Autodesk Inventor part; units mm, degrees
(part 3 of 18)
  ellipse E264 centre (-10091.4826, -10019.097) end of major axis (-10091.4826, -10024.058) minor radius 0.4679 (-10091.8131, -10015.5852) -> (-10091.9034, -10016.9265) ccw
  ellipse E265 centre (-10091.4826, -10019.097) end of major axis (-10091.4826, -10024.058) minor radius 0.4679 (-10091.9034, -10021.2675) -> (-10091.8131, -10022.6088) ccw
  spline S10 degree 3 poles (-10091.8131, -10022.6088) (-10091.7949, -10022.6489) (-10091.7591, -10022.7279) (-10091.7082, -10022.8453) (-10091.6607, -10022.9592) (-10091.617, -10023.0692) (-10091.5772, -10023.1748) (-10091.5414, -10023.2762) (-10091.5097, -10023.3737) (-10091.4825, -10023.4669) (-10091.4604, -10023.5539) (-10091.4445, -10023.6326) (-10091.435, -10023.7014) (-10091.4315, -10023.7595) (-10091.4337, -10023.8077) (-10091.4421, -10023.8464) (-10091.4557, -10023.8779) (-10091.4713, -10023.8914) (-10091.4786, -10023.8977) knots 0 0 0 0 0.096483 0.190064 0.280343 0.366935 0.449463 0.527566 0.602572 0.674179 0.740358 0.79923 0.84998 0.89243 0.926709 0.955226 0.979191 1 1 1 1
  spline S11 degree 3 poles (-10091.4786, -10014.2963) (-10091.4715, -10014.3024) (-10091.4562, -10014.3157) (-10091.4427, -10014.3469) (-10091.4344, -10014.3856) (-10091.4318, -10014.4331) (-10091.4346, -10014.4891) (-10091.4432, -10014.5537) (-10091.4576, -10014.6269) (-10091.4777, -10014.7086) (-10091.5032, -10014.7984) (-10091.5341, -10014.8954) (-10091.5699, -10014.9991) (-10091.6106, -10015.1085) (-10091.6559, -10015.2229) (-10091.7222, -10015.3831) (-10091.7765, -10015.5037) (-10091.8131, -10015.5852) knots 0 0 0 0 0.020314 0.043937 0.072556 0.107061 0.147904 0.195304 0.249736 0.311344 0.379674 0.454238 0.534533 0.62004 0.710199 0.804177 1 1 1 1
  ellipse E266 centre (-10090.9848, -10019.097) end of major axis (-10090.9848, -10013.636) minor radius 0.5151 (-10091.1548, -10013.9419) -> (-10091.4056, -10015.9471) ccw
  ellipse E267 centre (-10090.9848, -10019.097) end of major axis (-10090.9848, -10024.558) minor radius 0.5151 (-10091.4056, -10022.2469) -> (-10091.1548, -10024.252) ccw
  line L363 (-10091.2821, -10013.293) -> (-10089.4849, -10013.1227)
  spline S12 degree 3 poles (-10091.6874, -10014.3153) (-10091.6596, -10014.2332) (-10091.6029, -10014.0662) (-10091.5232, -10013.8583) (-10091.4546, -10013.6887) (-10091.3999, -10013.5584) (-10091.3424, -10013.4262) (-10091.3023, -10013.3377) (-10091.2821, -10013.293) knots 0 0 0 0 0.236217 0.480946 0.606817 0.735194 0.86621 1 1 1 1
  line L364 (-10091.612, -10015.111) -> (-10091.6874, -10014.3153)
  ellipse E268 centre (-10091.4826, -10016.4757) end of major axis (-10091.0145, -10021.4146) minor radius 0.0001 (-10091.8141, -10012.9784) -> (-10091.6876, -10014.3134) ccw
  ellipse E269 centre (-10091.4826, -10016.4757) end of major axis (-10091.9507, -10011.5369) minor radius 0.0001 (-10091.9507, -10011.5369) -> (-10091.9347, -10011.7067) ccw
  spline S13 degree 3 poles (-10091.9347, -10011.7067) (-10091.9147, -10011.6982) (-10091.8771, -10011.6824) (-10091.8201, -10011.6715) (-10091.7675, -10011.6743) (-10091.7211, -10011.6947) (-10091.6835, -10011.7317) (-10091.6548, -10011.7832) (-10091.6347, -10011.8485) (-10091.6229, -10011.9278) (-10091.6198, -10012.0211) (-10091.6249, -10012.128) (-10091.638, -10012.2477) (-10091.659, -10012.3786) (-10091.6876, -10012.5192) (-10091.7236, -10012.6679) (-10091.7657, -10012.8226) (-10091.7978, -10012.9269) (-10091.814, -10012.9798) knots 0 0 0 0 0.041849 0.07857 0.111147 0.141904 0.174268 0.211184 0.254599 0.305659 0.365519 0.434561 0.512207 0.59776 0.690456 0.789354 0.89303 1 1 1 1
  ellipse E270 centre (-10090.9848, -10016.4286) end of major axis (-10091.5002, -10010.9919) minor radius 0.0001 (-10091.5002, -10010.9919) -> (-10091.2821, -10013.293) ccw
  line L365 (-10091.9507, -10011.5369) -> (-10091.5002, -10010.9919)
  line L366 (-10089.85, -10010.8355) -> (-10091.5002, -10010.9919)
  ellipse E271 centre (-10092.0111, -10021.9287) end of major axis (-10092.4185, -10025.8225) minor radius 0.0003 (-10092.049, -10022.2884) -> (-10092.1813, -10023.5527) ccw
  ellipse E272 centre (-10092.2142, -10023.8677) end of major axis (-10092.1934, -10023.6687) minor radius 0 (-10092.2028, -10023.7589) -> (-10092.1934, -10023.6687) ccw
  line L367 (-10092.1934, -10023.6687) -> (-10092.1934, -10023.6687)
  ellipse E273 centre (-10092.1726, -10023.4698) end of major axis (-10092.1934, -10023.6687) minor radius 0 (-10092.1813, -10023.5527) -> (-10092.1934, -10023.6687) ccw
  ellipse E274 centre (-10092.0111, -10021.9287) end of major axis (-10092.3612, -10025.2755) minor radius 0.0002 (-10092.2028, -10023.7589) -> (-10092.3612, -10025.2755) ccw
  line L368 (-10092.3612, -10025.2755) -> (-10091.8251, -10025.3316)
  ellipse E275 centre (-10107.7253, -10020.2846) end of major axis (-10107.9605, -10022.5323) minor radius 0.0002 (-10107.9319, -10022.2582) -> (-10107.9605, -10022.5323) ccw
  line L369 (-10107.9605, -10022.5323) -> (-10106.0134, -10022.8287)
  line L370 (-10091.9034, -10017.347) -> (-10092.3628, -10017.347)
  ellipse E276 centre (-10092.3628, -10017.547) end of major axis (-10092.3628, -10017.347) minor radius 0.0208 (-10092.3628, -10017.347) -> (-10092.3817, -10017.4635) ccw
  ellipse E277 centre (-10092.0114, -10019.097) end of major axis (-10092.0114, -10023.012) minor radius 0.4074 (-10092.3817, -10017.4635) -> (-10092.3817, -10020.7304) ccw
  ellipse E278 centre (-10092.322, -10017.147) end of major axis (-10092.322, -10017.347) minor radius 0.0208 (-10092.322, -10017.347) -> (-10092.3046, -10017.2564) ccw
  ellipse E279 centre (-10092.322, -10021.047) end of major axis (-10092.322, -10020.847) minor radius 0.0208 (-10092.3046, -10020.9376) -> (-10092.322, -10020.847) ccw
  ellipse E280 centre (-10092.3628, -10020.647) end of major axis (-10092.3628, -10020.847) minor radius 0.0208 (-10092.3817, -10020.7304) -> (-10092.3628, -10020.847) ccw
  line L371 (-10092.3628, -10020.847) -> (-10091.9034, -10020.847)
  ellipse E281 centre (-10092.0114, -10019.097) end of major axis (-10092.0114, -10015.732) minor radius 0.3502 (-10092.0633, -10015.7691) -> (-10092.3046, -10017.2564) ccw
  ellipse E282 centre (-10092.0114, -10019.097) end of major axis (-10092.0114, -10022.462) minor radius 0.3502 (-10092.3046, -10020.9376) -> (-10092.0633, -10022.4248) ccw
  ellipse E283 centre (-10107.7256, -10019.097) end of major axis (-10107.7256, -10016.837) minor radius 0.2352 (-10107.9345, -10018.0589) -> (-10107.9345, -10020.1351) ccw
  ellipse E284 centre (-10092.1726, -10014.7242) end of major axis (-10092.1934, -10014.5253) minor radius 0 (-10092.1934, -10014.5253) -> (-10092.1813, -10014.6413) ccw
  ellipse E285 centre (-10092.0111, -10016.2653) end of major axis (-10091.6037, -10020.159) minor radius 0.0003 (-10092.1813, -10014.6412) -> (-10092.049, -10015.9055) ccw
  line L372 (-10092.1934, -10014.5252) -> (-10092.1934, -10014.5253)
  ellipse E286 centre (-10092.2142, -10014.3263) end of major axis (-10092.1934, -10014.5252) minor radius 0 (-10092.1934, -10014.5252) -> (-10092.2028, -10014.4351) ccw
  ellipse E287 centre (-10092.0111, -10016.2653) end of major axis (-10092.3612, -10012.9185) minor radius 0.0002 (-10092.3612, -10012.9185) -> (-10092.2028, -10014.4351) ccw
  line L373 (-10092.3612, -10012.9185) -> (-10091.8251, -10012.8624)
  ellipse E288 centre (-10107.7253, -10017.9094) end of major axis (-10107.9605, -10015.6616) minor radius 0.0002 (-10107.9605, -10015.6616) -> (-10107.9319, -10015.9358) ccw
  line L374 (-10107.9605, -10015.6616) -> (-10106.0134, -10015.3653)
  ellipse E289 centre (-10105.7572, -10020.6362) end of major axis (-10106.0195, -10022.8809) minor radius 0.0001 (-10105.931, -10022.1228) -> (-10106.0195, -10022.8809) ccw
  line L375 (-10106.0195, -10022.8809) -> (-10094.287, -10024.8118)
  line L376 (-10093.9901, -10024.8606) -> (-10092.3462, -10025.1312)
  ellipse E290 centre (-10090.0644, -10019.097) end of major axis (-10090.0644, -10023.012) minor radius 0.4538 (-10090.5105, -10018.3786) -> (-10090.5126, -10018.4825) ccw
  ellipse E291 centre (-10090.0644, -10019.097) end of major axis (-10090.0644, -10023.012) minor radius 0.4538 (-10090.5165, -10018.7563) -> (-10090.5159, -10019.4926) ccw
  ellipse E292 centre (-10090.0644, -10019.097) end of major axis (-10090.0644, -10023.012) minor radius 0.4538 (-10090.5126, -10019.7115) -> (-10090.5105, -10019.8154) ccw
  ellipse E293 centre (-10105.7579, -10019.097) end of major axis (-10105.7579, -10016.837) minor radius 0.262 (-10105.9293, -10017.388) -> (-10105.9293, -10020.806) ccw
  ellipse E294 centre (-10105.7572, -10017.5578) end of major axis (-10106.0195, -10015.313) minor radius 0.0001 (-10106.0195, -10015.313) -> (-10105.931, -10016.0712) ccw
  line L377 (-10106.0195, -10015.313) -> (-10094.287, -10013.3822)
  line L378 (-10093.9901, -10013.3333) -> (-10092.3462, -10013.0628)
  ellipse E295 centre (-10110.6856, -10019.8981) end of major axis (-10110.6663, -10019.694) minor radius 0 (-10110.6663, -10019.694) -> (-10110.6896, -10019.9398) ccw
  ellipse E296 centre (-10110.2516, -10019.9392) end of major axis (-10110.3681, -10021.1687) minor radius 0 (-10110.2842, -10020.2826) -> (-10110.3681, -10021.1687) ccw
  line L379 (-10110.3681, -10021.1687) -> (-10109.8175, -10021.2209)
  arc A0 (-10110.6961, -10020.2655) -> (-10110.3681, -10021.1687) centre (-10108.7751, -10020.0791) ccw
  arc A1 (-10110.6416, -10019.5881) -> (-10110.6663, -10019.694) centre (-10108.7751, -10020.0791) ccw
  ellipse E297 centre (-10093.9714, -10021.4823) end of major axis (-10094.3409, -10025.3799) minor radius 0 (-10094.032, -10022.1204) -> (-10094.1256, -10023.1082) ccw
  ellipse E298 centre (-10092.9759, -10021.5767) end of major axis (-10093.3453, -10025.4742) minor radius 0 (-10092.9997, -10021.8271) -> (-10093.1301, -10023.2026) ccw
  line L380 (-10094.1366, -10023.2243) -> (-10094.1366, -10023.2243)
  line L381 (-10093.1411, -10023.3186) -> (-10093.1411, -10023.3187)
  ellipse E299 centre (-10093.9714, -10021.4823) end of major axis (-10094.289, -10024.8323) minor radius 0 (-10094.1451, -10023.3145) -> (-10094.289, -10024.8323) ccw
  ellipse E300 centre (-10092.9759, -10021.5767) end of major axis (-10093.2934, -10024.9267) minor radius 0 (-10093.1496, -10023.4089) -> (-10093.2706, -10024.6854) ccw
  line L382 (-10094.289, -10024.8323) -> (-10093.9901, -10024.8606)
  ellipse E301 centre (-10109.7009, -10019.9914) end of major axis (-10109.9142, -10022.2413) minor radius 0 (-10109.8038, -10021.0763) -> (-10109.9142, -10022.2413) ccw
  line L383 (-10109.9142, -10022.2413) -> (-10107.9592, -10022.5194)
  ellipse E302 centre (-10110.2517, -10019.097) end of major axis (-10110.2517, -10017.862) minor radius 0.1165 (-10110.2842, -10017.9113) -> (-10110.2842, -10020.2827) ccw
  arc A2 (-10110.6943, -10019.3011) -> (-10110.4368, -10020.0787) centre (-10108.7751, -10019.097) ccw
  arc A3 (-10110.4368, -10018.1153) -> (-10110.6943, -10018.8928) centre (-10108.7751, -10019.097) ccw
  ellipse E303 centre (-10093.2944, -10017.547) end of major axis (-10093.2944, -10017.347) minor radius 0.0189 (-10093.2944, -10017.347) -> (-10093.3115, -10017.4635) ccw
  line L384 (-10093.2944, -10017.347) -> (-10094.2899, -10017.347)
  ellipse E304 centre (-10094.2899, -10017.547) end of major axis (-10094.2899, -10017.347) minor radius 0.0189 (-10094.2899, -10017.347) -> (-10094.307, -10017.4635) ccw
  ellipse E305 centre (-10093.9714, -10019.097) end of major axis (-10093.9714, -10023.012) minor radius 0.3693 (-10094.307, -10017.4635) -> (-10094.307, -10020.7304) ccw
  ellipse E306 centre (-10092.9759, -10019.097) end of major axis (-10092.9759, -10023.012) minor radius 0.3693 (-10093.3115, -10017.4635) -> (-10093.3115, -10020.7304) ccw
  ellipse E307 centre (-10094.2529, -10017.147) end of major axis (-10094.2529, -10017.347) minor radius 0.0189 (-10094.2529, -10017.347) -> (-10094.2371, -10017.2564) ccw
  ellipse E308 centre (-10094.2529, -10021.047) end of major axis (-10094.2529, -10020.847) minor radius 0.0189 (-10094.2371, -10020.9376) -> (-10094.2529, -10020.847) ccw
  ellipse E309 centre (-10094.2899, -10020.647) end of major axis (-10094.2899, -10020.847) minor radius 0.0189 (-10094.307, -10020.7304) -> (-10094.2899, -10020.847) ccw
  ellipse E310 centre (-10093.2944, -10020.647) end of major axis (-10093.2944, -10020.847) minor radius 0.0189 (-10093.3115, -10020.7304) -> (-10093.2944, -10020.847) ccw
  line L385 (-10094.2899, -10020.847) -> (-10093.2944, -10020.847)
  ellipse E311 centre (-10093.2574, -10017.147) end of major axis (-10093.2574, -10017.347) minor radius 0.0189 (-10093.2574, -10017.347) -> (-10093.2416, -10017.2564) ccw
  line L386 (-10093.2574, -10017.347) -> (-10093.2944, -10017.347)
  ellipse E312 centre (-10093.2574, -10021.047) end of major axis (-10093.2574, -10020.847) minor radius 0.0189 (-10093.2416, -10020.9376) -> (-10093.2574, -10020.847) ccw
  line L387 (-10093.2944, -10020.847) -> (-10093.2574, -10020.847)
  ellipse E313 centre (-10093.9714, -10019.097) end of major axis (-10093.9714, -10015.732) minor radius 0.3174 (-10094.0535, -10015.8464) -> (-10094.2371, -10017.2564) ccw
  ellipse E314 centre (-10093.9714, -10019.097) end of major axis (-10093.9714, -10022.462) minor radius 0.3174 (-10094.2371, -10020.9376) -> (-10094.0535, -10022.3476) ccw
  ellipse E315 centre (-10092.9759, -10019.097) end of major axis (-10092.9759, -10022.462) minor radius 0.3174 (-10093.0508, -10022.3668) -> (-10093.0151, -10022.4363) ccw
  ellipse E316 centre (-10092.9759, -10019.097) end of major axis (-10092.9759, -10015.732) minor radius 0.3174 (-10093.2416, -10020.9376) -> (-10093.1078, -10022.1578) ccw
  ellipse E317 centre (-10092.9759, -10019.097) end of major axis (-10092.9759, -10015.732) minor radius 0.3174 (-10093.1078, -10016.0361) -> (-10093.2416, -10017.2564) ccw
  ellipse E318 centre (-10092.9759, -10019.097) end of major axis (-10092.9759, -10015.732) minor radius 0.3174 (-10093.0151, -10015.7577) -> (-10093.0508, -10015.8271) ccw
  ellipse E319 centre (-10109.701, -10019.097) end of major axis (-10109.701, -10016.837) minor radius 0.2132 (-10109.8038, -10017.1174) -> (-10109.8038, -10021.0766) ccw
  ellipse E320 centre (-10110.6856, -10018.2959) end of major axis (-10110.6663, -10018.5) minor radius 0 (-10110.6896, -10018.2541) -> (-10110.6663, -10018.5) ccw
  ellipse E321 centre (-10110.2516, -10018.2548) end of major axis (-10110.3681, -10017.0253) minor radius 0 (-10110.3681, -10017.0253) -> (-10110.2842, -10017.9114) ccw
  line L388 (-10110.3681, -10017.0253) -> (-10109.8175, -10016.9731)
  arc A4 (-10110.6663, -10018.5) -> (-10110.6416, -10018.6058) centre (-10108.7751, -10018.1148) ccw
  arc A5 (-10110.3681, -10017.0253) -> (-10110.6961, -10017.9284) centre (-10108.7751, -10018.1148) ccw
  ellipse E322 centre (-10093.9714, -10016.7117) end of major axis (-10093.602, -10020.6092) minor radius 0 (-10094.1256, -10015.0852) -> (-10094.032, -10016.073) ccw
  ellipse E323 centre (-10092.9759, -10016.6173) end of major axis (-10092.6065, -10020.5148) minor radius 0 (-10093.1301, -10014.9909) -> (-10092.9997, -10016.3663) ccw
  line L389 (-10094.1366, -10014.9697) -> (-10094.1366, -10014.9697)
  line L390 (-10093.1411, -10014.8753) -> (-10093.1411, -10014.8753)
  ellipse E324 centre (-10093.9714, -10016.7117) end of major axis (-10094.289, -10013.3617) minor radius 0 (-10094.289, -10013.3617) -> (-10094.1451, -10014.8796) ccw
  ellipse E325 centre (-10092.9759, -10016.6173) end of major axis (-10093.2934, -10013.2673) minor radius 0 (-10093.2706, -10013.5086) -> (-10093.1496, -10014.7851) ccw
  line L391 (-10094.289, -10013.3617) -> (-10093.9901, -10013.3333)
  ellipse E326 centre (-10109.7009, -10018.2026) end of major axis (-10109.9142, -10015.9527) minor radius 0 (-10109.9142, -10015.9527) -> (-10109.8038, -10017.1177) ccw
  line L392 (-10109.9142, -10015.9527) -> (-10107.9592, -10015.6746)
  line L393 (-10057.5, -10011.9318) -> (-10059.2152, -10012.5974)
  line L394 (-10057.5, -10009.857) -> (-10059.3806, -10010.3993)
  line L395 (-10057.5, -10028.891) -> (-10059.5192, -10028.9931)
  line L396 (-10057.5, -10026.8208) -> (-10059.4509, -10026.7182)
  line L397 (-10058.1625, -10011.9763) -> (-10059.2627, -10012.2094)
  line L398 (-10058.2161, -10009.8452) -> (-10059.471, -10009.9867)
  line L399 (-10058.2161, -10028.3488) -> (-10059.471, -10028.2072)
  line L400 (-10058.1625, -10026.2177) -> (-10059.2627, -10025.9845)
  line L401 (-10057.5, -10011.3732) -> (-10059.4509, -10011.4758)
  line L402 (-10057.5, -10009.3029) -> (-10059.5002, -10009.2018)
  line L403 (-10057.5, -10028.3369) -> (-10059.3884, -10027.7924)
  line L404 (-10057.5, -10026.2622) -> (-10059.2152, -10025.5966)
  line L405 (-10058.9107, -10011.6972) -> (-10059.3563, -10011.7799)
  line L406 (-10058.8961, -10009.5113) -> (-10059.5174, -10009.572)
  line L407 (-10058.8961, -10028.6826) -> (-10059.5174, -10028.622)
  line L408 (-10058.9107, -10026.4967) -> (-10059.3563, -10026.414)
  ellipse E327 centre (-10072.7505, -10029.5199) end of major axis (-10072.9258, -10029.5933) minor radius 0.1721 (-10072.7587, -10029.6947) -> (-10072.5839, -10029.5888) ccw
  ellipse E328 centre (-10072.726, -10029.5786) end of major axis (-10072.5507, -10029.5052) minor radius 0.1721 (-10072.6178, -10029.7139) -> (-10072.564, -10029.6557) ccw
  ellipse E329 centre (-10069.9466, -10029.5086) end of major axis (-10070.1219, -10029.5819) minor radius 0.1721 (-10070.0985, -10029.6208) -> (-10070.0788, -10029.641) ccw
  ellipse E330 centre (-10072.7276, -10029.77) end of major axis (-10072.5378, -10029.7788) minor radius 0.074 (-10072.5404, -10029.7652) -> (-10072.7587, -10029.6957) ccw
  ellipse E331 centre (-10072.7341, -10029.908) end of major axis (-10072.5443, -10029.9168) minor radius 0.074 (-10072.5468, -10029.9032) -> (-10072.7652, -10029.8337) ccw
  ellipse E332 centre (-10069.9548, -10029.8379) end of major axis (-10070.1445, -10029.8291) minor radius 0.074 (-10069.9859, -10029.7636) -> (-10070.142, -10029.8427) ccw
  ellipse E333 centre (-10069.9712, -10029.4499) end of major axis (-10070.1465, -10029.5233) minor radius 0.1721 (-10070.1293, -10029.5541) -> (-10069.9794, -10029.6247) ccw
  ellipse E334 centre (-10069.9483, -10029.6999) end of major axis (-10070.1381, -10029.6911) minor radius 0.074 (-10069.9794, -10029.6256) -> (-10070.1381, -10029.6911) ccw
  line L409 (-10070.1381, -10029.6911) -> (-10070.1445, -10029.8291)
  line L410 (-10072.5313, -10029.416) -> (-10072.5356, -10029.507)
  line L411 (-10072.5594, -10029.4332) -> (-10072.5539, -10029.3142)
  line L412 (-10070.289, -10028.8289) -> (-10070.7236, -10028.8398)
  line L413 (-10072.1226, -10028.8751) -> (-10072.3193, -10028.88)
  line L414 (-10072.4473, -10030.1409) -> (-10072.5468, -10029.9032)
  line L415 (-10072.5404, -10029.7652) -> (-10072.4857, -10029.8959)
  line L416 (-10070.142, -10029.8427) -> (-10070.0999, -10029.9432)
  line L417 (-10070.1967, -10030.1641) -> (-10072.227, -10030.2153)
  line L418 (-10070.1488, -10029.247) -> (-10070.1526, -10029.3284)
  line L419 (-10072.2205, -10030.0773) -> (-10070.1902, -10030.0261)
  line L420 (-10072.3438, -10028.8214) -> (-10072.1091, -10028.8155)
  line L421 (-10071.0809, -10028.7896) -> (-10070.3135, -10028.7702)
  ellipse E335 centre (-10074.1058, -10029.6134) end of major axis (-10074.281, -10029.6867) minor radius 0.1721 (-10074.281, -10029.6867) -> (-10074.2379, -10029.7458) ccw
  ellipse E336 centre (-10068.5668, -10029.4738) end of major axis (-10068.3916, -10029.4004) minor radius 0.1721 (-10068.4586, -10029.6091) -> (-10068.4439, -10029.5974) ccw
  ellipse E337 centre (-10068.5914, -10029.4151) end of major axis (-10068.7667, -10029.4885) minor radius 0.1721 (-10068.5996, -10029.5899) -> (-10068.4595, -10029.5304) ccw
  ellipse E338 centre (-10074.1303, -10029.5547) end of major axis (-10074.3056, -10029.6281) minor radius 0.1721 (-10074.3109, -10029.6133) -> (-10074.1385, -10029.7295) ccw
  line L422 (-10074.281, -10029.6867) -> (-10074.3056, -10029.6281)
  line L423 (-10068.3786, -10029.4474) -> (-10068.3312, -10028.4341)
  line L424 (-10068.5996, -10029.5899) -> (-10069.9794, -10029.6247)
  line L425 (-10068.386, -10029.0227) -> (-10068.4024, -10029.3736)
  line L426 (-10074.3076, -10029.3456) -> (-10074.3053, -10029.297)
  line L427 (-10072.7587, -10029.6947) -> (-10074.1385, -10029.7295)
  ellipse E339 centre (-10070.2971, -10029.0037) end of major axis (-10070.1219, -10028.9303) minor radius 0.1721 (-10070.1745, -10028.8637) -> (-10070.289, -10028.8289) ccw
  ellipse E340 centre (-10072.3274, -10029.0549) end of major axis (-10072.1522, -10028.9815) minor radius 0.1721 (-10072.3193, -10028.88) -> (-10072.371, -10028.8881) ccw
  ellipse E341 centre (-10070.2278, -10030.0898) end of major axis (-10070.038, -10030.0987) minor radius 0.074 (-10070.1967, -10030.1641) -> (-10070.0949, -10030.148) ccw
  ellipse E342 centre (-10072.2581, -10030.141) end of major axis (-10072.4479, -10030.1321) minor radius 0.074 (-10072.437, -10030.1586) -> (-10072.227, -10030.2153) ccw
  ellipse E343 centre (-10072.352, -10028.9962) end of major axis (-10072.5272, -10029.0696) minor radius 0.1721 (-10072.3438, -10028.8214) -> (-10072.4426, -10028.8494) ccw
  ellipse E344 centre (-10070.3217, -10028.945) end of major axis (-10070.1464, -10028.8717) minor radius 0.1721 (-10070.1723, -10028.8299) -> (-10070.3135, -10028.7702) ccw
  ellipse E345 centre (-10070.2213, -10029.9518) end of major axis (-10070.4111, -10029.9429) minor radius 0.074 (-10070.1902, -10030.0261) -> (-10070.1092, -10030.016) ccw
  ellipse E346 centre (-10072.2516, -10030.003) end of major axis (-10072.4414, -10029.9941) minor radius 0.074 (-10072.2933, -10030.0736) -> (-10072.2205, -10030.0773) ccw
  line L428 (-10072.7652, -10029.8337) -> (-10074.145, -10029.8684)
  line L429 (-10074.3011, -10029.9474) -> (-10074.2237, -10030.1324)
  line L430 (-10068.2006, -10030.2453) -> (-10068.3877, -10029.7984)
  line L431 (-10068.606, -10029.7289) -> (-10069.9859, -10029.7636)
  line L432 (-10072.7587, -10029.6957) -> (-10074.1385, -10029.7304)
  line L433 (-10068.5996, -10029.5909) -> (-10069.9794, -10029.6256)
  line L434 (-10068.0244, -10030.5129) -> (-10068.3812, -10029.6604)
  ellipse E347 centre (-10074.1139, -10029.9427) end of major axis (-10074.3037, -10029.9339) minor radius 0.074 (-10074.145, -10029.8684) -> (-10074.3011, -10029.9474) ccw
  ellipse E348 centre (-10068.5749, -10029.8032) end of major axis (-10068.3852, -10029.812) minor radius 0.074 (-10068.3877, -10029.7984) -> (-10068.606, -10029.7289) ccw
  ellipse E349 centre (-10074.1074, -10029.8047) end of major axis (-10074.2972, -10029.7959) minor radius 0.074 (-10074.1385, -10029.7304) -> (-10074.2972, -10029.7959) ccw
  ellipse E350 centre (-10068.5685, -10029.6652) end of major axis (-10068.3787, -10029.674) minor radius 0.074 (-10068.3812, -10029.6604) -> (-10068.5996, -10029.5909) ccw
  line L435 (-10074.3037, -10029.9339) -> (-10074.2972, -10029.7959)
  line L436 (-10067.943, -10029.7444) -> (-10067.9727, -10030.3807)
  line L437 (-10067.9482, -10030.4393) -> (-10067.9157, -10029.743)
  ellipse E351 centre (-10068.0137, -10030.2829) end of major axis (-10068.0074, -10030.5328) minor radius 0.0419 (-10068.0244, -10030.5129) -> (-10067.9727, -10030.3807) ccw
  ellipse E352 centre (-10068.0137, -10030.2829) end of major axis (-10068.0036, -10030.6828) minor radius 0.067 (-10068.0104, -10030.6809) -> (-10067.9482, -10030.4393) ccw
  line L438 (-10068.0095, -10030.6829) -> (-10068.0036, -10030.6828)
  line L439 (-10072.5875, -10009.656) -> (-10072.5979, -10009.3751)
  line L440 (-10070.348, -10009.5238) -> (-10071.6175, -10009.6568)
  ellipse E353 centre (-10074.1798, -10009.4887) end of major axis (-10074.3681, -10009.5136) minor radius 0.1017 (-10074.2752, -10009.4093) -> (-10074.3686, -10009.5084) ccw
  line L441 (-10074.3686, -10009.5084) -> (-10074.3647, -10009.6117)
  line L442 (-10068.3867, -10009.4202) -> (-10068.3977, -10009.1255)
  line L443 (-10068.3981, -10009.1151) -> (-10068.4006, -10009.0465)
  line L444 (-10068.3679, -10009.6071) -> (-10068.3718, -10009.5008)
  ellipse E354 centre (-10070.3518, -10009.4219) end of major axis (-10070.1634, -10009.3969) minor radius 0.1017 (-10070.348, -10009.5238) -> (-10070.1709, -10009.4343) ccw
  ellipse E355 centre (-10072.3987, -10009.6362) end of major axis (-10072.5871, -10009.6611) minor radius 0.1017 (-10072.5875, -10009.656) -> (-10072.5875, -10009.6563) ccw
  line L445 (-10074.3483, -10028.4712) -> (-10074.3484, -10028.5612)
  line L446 (-10068.3859, -10028.8059) -> (-10068.3858, -10028.7663)
  line L447 (-10068.3855, -10028.5773) -> (-10068.3852, -10028.3465)
  line L448 (-10068.5739, -10028.2536) -> (-10069.2672, -10028.181)
  line L449 (-10068.3691, -10028.6827) -> (-10068.3689, -10028.6135)
  ellipse E356 centre (-10068.574, -10028.3267) end of major axis (-10068.3854, -10028.3499) minor radius 0.0727 (-10068.3852, -10028.3465) -> (-10068.5739, -10028.2536) ccw
  line L450 (-10070.1541, -10028.3154) -> (-10070.1542, -10028.3591)
  ellipse E357 centre (-10074.3034, -10028.1944) end of major axis (-10074.3451, -10028.5922) minor radius 0.0171 (-10074.3484, -10028.5612) -> (-10074.3451, -10028.5922) ccw
  line L451 (-10074.3451, -10028.5922) -> (-10074.3402, -10028.5927)
  line L452 (-10068.0255, -10007.6833) -> (-10067.9929, -10008.0725)
  line L453 (-10067.9312, -10008.4502) -> (-10068.0025, -10007.6018)
  ellipse E358 centre (-10068.2128, -10007.6785) end of major axis (-10068.03, -10007.7303) minor radius 0.1568 (-10068.0255, -10007.6833) -> (-10068.0605, -10007.5988) ccw
  ellipse E359 centre (-10068.1897, -10007.597) end of major axis (-10068.0069, -10007.6488) minor radius 0.1568 (-10068.0025, -10007.6018) -> (-10068.0393, -10007.515) ccw
  line L454 (-10074.2957, -10008.4229) -> (-10074.3046, -10008.4542)
  line L455 (-10068.3912, -10008.6032) -> (-10068.2666, -10008.1635)
  line L456 (-10068.3471, -10008.6108) -> (-10068.0452, -10007.5447)
  line L457 (-10072.5503, -10008.4984) -> (-10072.4611, -10008.1833)
  line L458 (-10072.2446, -10008.0848) -> (-10070.2143, -10008.136)
  ellipse E360 centre (-10072.5221, -10008.8341) end of major axis (-10072.512, -10008.4342) minor radius 0.067 (-10072.5503, -10008.4984) -> (-10072.5838, -10008.7233) ccw
  line L459 (-10072.5496, -10009.4566) -> (-10072.5782, -10009.1162)
  ellipse E361 centre (-10072.5221, -10008.8341) end of major axis (-10072.5284, -10009.084) minor radius 0.0419 (-10072.5643, -10008.8499) -> (-10072.5611, -10008.964) ccw
  line L460 (-10072.4954, -10008.4678) -> (-10072.5139, -10008.5332)
  ellipse E362 centre (-10070.1173, -10008.8947) end of major axis (-10070.1274, -10009.2946) minor radius 0.067 (-10070.1482, -10008.5689) -> (-10070.1825, -10008.8444) ccw
  line L461 (-10072.3247, -10009.5537) -> (-10072.0713, -10009.56)
  ellipse E363 centre (-10072.2738, -10008.188) end of major axis (-10072.4631, -10008.2039) minor radius 0.1025 (-10072.2446, -10008.0848) -> (-10072.4611, -10008.1833) ccw
  ellipse E364 centre (-10070.2435, -10008.2392) end of major axis (-10070.4328, -10008.2551) minor radius 0.1025 (-10070.0994, -10008.1639) -> (-10070.2143, -10008.136) ccw
  ellipse E365 centre (-10072.3381, -10009.3942) end of major axis (-10072.5209, -10009.3424) minor radius 0.1568 (-10072.3894, -10009.5425) -> (-10072.3247, -10009.5537) ccw
  ellipse E366 centre (-10072.3612, -10009.4757) end of major axis (-10072.1784, -10009.5275) minor radius 0.1568 (-10072.5392, -10009.5108) -> (-10072.4498, -10009.608) ccw
  line L462 (-10068.3438, -10009.7619) -> (-10068.3687, -10009.465)
  line L463 (-10068.3966, -10009.133) -> (-10068.4015, -10009.0747)
  ellipse E367 centre (-10068.363, -10008.9389) end of major axis (-10068.3567, -10008.689) minor radius 0.0419 (-10068.4046, -10008.9298) -> (-10068.4015, -10009.0747) ccw
  ellipse E368 centre (-10074.2764, -10008.7899) end of major axis (-10074.2865, -10009.1898) minor radius 0.067 (-10074.3046, -10008.4542) -> (-10074.3424, -10008.7578) ccw
  ellipse E369 centre (-10068.363, -10008.9389) end of major axis (-10068.3731, -10009.3388) minor radius 0.067 (-10068.3912, -10008.6032) -> (-10068.4193, -10008.7679) ccw
  ellipse E370 centre (-10068.2324, -10007.54) end of major axis (-10068.0431, -10007.5241) minor radius 0.1025 (-10068.0452, -10007.5447) -> (-10068.043, -10007.5255) ccw
  line L464 (-10067.9879, -10010.0299) -> (-10068.0005, -10010.0742)
  ellipse E371 centre (-10072.7175, -10029.8579) end of major axis (-10072.8916, -10029.934) minor radius 0.169 (-10072.7233, -10030.0302) -> (-10072.5613, -10029.9399) ccw
  ellipse E372 centre (-10072.69, -10029.9208) end of major axis (-10072.5159, -10029.8447) minor radius 0.169 (-10072.5774, -10030.049) -> (-10072.5311, -10029.9984) ccw
  ellipse E373 centre (-10072.6886, -10030.1107) end of major axis (-10072.4987, -10030.1171) minor radius 0.0799 (-10072.5019, -10030.1013) -> (-10072.7233, -10030.0311) ccw
  ellipse E374 centre (-10072.6932, -10030.2467) end of major axis (-10072.5033, -10030.2531) minor radius 0.0799 (-10072.5065, -10030.2373) -> (-10072.7279, -10030.1671) ccw
  ellipse E375 centre (-10069.9221, -10030.1066) end of major axis (-10070.112, -10030.1002) minor radius 0.0799 (-10069.9569, -10030.027) -> (-10070.1088, -10030.116) ccw
  ellipse E376 centre (-10069.9464, -10029.7178) end of major axis (-10070.1205, -10029.7939) minor radius 0.169 (-10070.0706, -10029.8561) -> (-10069.9523, -10029.8901) ccw
  ellipse E377 centre (-10069.9175, -10029.9706) end of major axis (-10070.1074, -10029.9642) minor radius 0.0799 (-10069.9523, -10029.891) -> (-10070.1074, -10029.9642) ccw
  line L465 (-10070.1074, -10029.9642) -> (-10070.112, -10030.1002)
  line L466 (-10072.4989, -10029.7812) -> (-10072.5015, -10029.858)
  line L467 (-10072.5289, -10029.7927) -> (-10072.5263, -10029.7174)
  line L468 (-10070.2694, -10029.1204) -> (-10070.6271, -10029.1385)
  line L469 (-10072.1017, -10029.2131) -> (-10072.2937, -10029.2228)
  line L470 (-10072.393, -10030.497) -> (-10072.5065, -10030.2373)
  line L471 (-10072.5019, -10030.1013) -> (-10072.3884, -10030.3609)
  line L472 (-10072.1076, -10031.1504) -> (-10072.2138, -10030.9074)
  line L473 (-10072.0618, -10030.8184) -> (-10070.0376, -10030.7161)
  line L474 (-10069.8161, -10030.7862) -> (-10069.71, -10031.0292)
  line L475 (-10070.1088, -10030.116) -> (-10069.9954, -10030.3757)
  line L476 (-10070.1473, -10030.4648) -> (-10072.1716, -10030.5671)
  line L477 (-10070.1302, -10029.6421) -> (-10070.1313, -10029.673)
  line L478 (-10072.167, -10030.4311) -> (-10070.1427, -10030.3288)
  ellipse E378 centre (-10072.0954, -10030.7877) end of major axis (-10072.0752, -10031.1872) minor radius 0.0715 (-10072.1076, -10031.1504) -> (-10072.0222, -10030.9552) ccw
  line L479 (-10072.0175, -10030.8162) -> (-10072.0222, -10030.9552)
  line L480 (-10072.0496, -10030.8924) -> (-10072.0477, -10030.8348)
  ellipse E379 centre (-10072.0954, -10030.7877) end of major axis (-10072.0828, -10031.0374) minor radius 0.0447 (-10072.103, -10031.0144) -> (-10072.0496, -10030.8924) ccw
  line L481 (-10072.1771, -10030.8448) -> (-10072.103, -10031.0144)
  ellipse E380 centre (-10069.6977, -10030.6665) end of major axis (-10069.6775, -10031.066) minor radius 0.0715 (-10069.71, -10031.0292) -> (-10069.6775, -10031.066) ccw
  line L482 (-10072.3211, -10029.1599) -> (-10072.0378, -10029.1456)
  line L483 (-10070.6475, -10029.0753) -> (-10070.2969, -10029.0576)
  ellipse E381 centre (-10074.0657, -10029.9903) end of major axis (-10074.2399, -10030.0664) minor radius 0.169 (-10074.2399, -10030.0664) -> (-10074.1999, -10030.1205) ccw
  ellipse E382 centre (-10068.5433, -10029.7111) end of major axis (-10068.3692, -10029.6351) minor radius 0.169 (-10068.3578, -10029.7165) -> (-10068.3566, -10029.7017) ccw
  ellipse E383 centre (-10068.5707, -10029.6483) end of major axis (-10068.7448, -10029.7243) minor radius 0.169 (-10068.3852, -10029.6532) -> (-10068.384, -10029.6388) ccw
  ellipse E384 centre (-10068.5707, -10029.6483) end of major axis (-10068.7448, -10029.7243) minor radius 0.169 (-10068.5766, -10029.8206) -> (-10068.5035, -10029.8033) ccw
  ellipse E385 centre (-10074.0932, -10029.9275) end of major axis (-10074.2673, -10030.0035) minor radius 0.169 (-10074.2698, -10029.9974) -> (-10074.099, -10030.0998) ccw
  line L484 (-10074.2399, -10030.0664) -> (-10074.2673, -10030.0035)
  line L485 (-10068.3566, -10029.7017) -> (-10068.356, -10029.685)
  line L486 (-10068.3509, -10029.5331) -> (-10068.3139, -10028.4395)
  line L487 (-10068.5766, -10029.8206) -> (-10069.9523, -10029.8901)
  line L488 (-10068.3748, -10029.3677) -> (-10068.3776, -10029.4503)
  line L489 (-10068.3833, -10029.6184) -> (-10068.384, -10029.6388)
  line L490 (-10074.274, -10029.7626) -> (-10074.2734, -10029.7447)
  line L491 (-10072.7233, -10030.0302) -> (-10074.099, -10030.0998)
  ellipse E386 centre (-10070.2752, -10029.2927) end of major axis (-10070.1011, -10029.2167) minor radius 0.169 (-10070.189, -10029.1334) -> (-10070.2694, -10029.1204) ccw
  ellipse E387 centre (-10072.2995, -10029.395) end of major axis (-10072.1254, -10029.319) minor radius 0.169 (-10072.2937, -10029.2228) -> (-10072.3389, -10029.2301) ccw
  ellipse E388 centre (-10072.0271, -10030.898) end of major axis (-10072.2169, -10030.8916) minor radius 0.0799 (-10072.0618, -10030.8184) -> (-10072.2138, -10030.9074) ccw
  ellipse E389 centre (-10070.0028, -10030.7957) end of major axis (-10069.8129, -10030.8021) minor radius 0.0799 (-10069.8161, -10030.7862) -> (-10070.0376, -10030.7161) ccw
  ellipse E390 centre (-10070.1821, -10030.3852) end of major axis (-10069.9922, -10030.3916) minor radius 0.0799 (-10070.1473, -10030.4648) -> (-10069.9954, -10030.3757) ccw
  ellipse E391 centre (-10072.2063, -10030.4875) end of major axis (-10072.3962, -10030.4811) minor radius 0.0799 (-10072.393, -10030.497) -> (-10072.1716, -10030.5671) ccw
  ellipse E392 centre (-10072.3269, -10029.3322) end of major axis (-10072.501, -10029.4083) minor radius 0.169 (-10072.3211, -10029.1599) -> (-10072.3606, -10029.1658) ccw
  ellipse E393 centre (-10070.3027, -10029.2299) end of major axis (-10070.4768, -10029.3059) minor radius 0.169 (-10070.178, -10029.092) -> (-10070.2969, -10029.0576) ccw
  ellipse E394 centre (-10070.1775, -10030.2492) end of major axis (-10070.3674, -10030.2427) minor radius 0.0799 (-10070.1427, -10030.3288) -> (-10070.0274, -10030.3024) ccw
  ellipse E395 centre (-10072.2017, -10030.3515) end of major axis (-10072.3916, -10030.3451) minor radius 0.0799 (-10072.3884, -10030.3609) -> (-10072.167, -10030.4311) ccw
  line L492 (-10072.7279, -10030.1671) -> (-10074.1036, -10030.2367)
  line L493 (-10074.2556, -10030.3257) -> (-10073.8568, -10031.2388)
  line L494 (-10067.9609, -10030.9407) -> (-10068.3597, -10030.0276)
  line L495 (-10068.5812, -10029.9575) -> (-10069.9569, -10030.027)
  line L496 (-10072.7233, -10030.0311) -> (-10074.099, -10030.1007)
  line L497 (-10068.5766, -10029.8215) -> (-10069.9523, -10029.891)
  line L498 (-10067.9563, -10030.8047) -> (-10068.3551, -10029.8916)
  ellipse E396 centre (-10074.0689, -10030.3162) end of major axis (-10074.2588, -10030.3098) minor radius 0.0799 (-10074.1036, -10030.2367) -> (-10074.2556, -10030.3257) ccw
  ellipse E397 centre (-10068.5464, -10030.0371) end of major axis (-10068.3565, -10030.0435) minor radius 0.0799 (-10068.3597, -10030.0276) -> (-10068.5812, -10029.9575) ccw
  ellipse E398 centre (-10074.0643, -10030.1802) end of major axis (-10074.2542, -10030.1738) minor radius 0.0799 (-10074.099, -10030.1007) -> (-10074.2542, -10030.1738) ccw
  ellipse E399 centre (-10068.5418, -10029.901) end of major axis (-10068.3519, -10029.9075) minor radius 0.0799 (-10068.3551, -10029.8916) -> (-10068.5766, -10029.8215) ccw
  line L499 (-10074.2588, -10030.3098) -> (-10074.2542, -10030.1738)
  line L500 (-10067.871, -10029.7408) -> (-10067.9029, -10030.6828)
  line L501 (-10067.8754, -10030.7456) -> (-10067.8414, -10029.7393)
  ellipse E400 centre (-10067.9486, -10030.5781) end of major axis (-10067.936, -10030.8277) minor radius 0.0447 (-10067.9563, -10030.8047) -> (-10067.9029, -10030.6828) ccw
  ellipse E401 centre (-10073.8445, -10030.8761) end of major axis (-10073.8243, -10031.2756) minor radius 0.0715 (-10073.8568, -10031.2388) -> (-10073.8243, -10031.2756) ccw
  ellipse E402 centre (-10067.9486, -10030.5781) end of major axis (-10067.9284, -10030.9775) minor radius 0.0715 (-10067.9609, -10030.9407) -> (-10067.8754, -10030.7456) ccw
  line L502 (-10073.8243, -10031.2756) -> (-10072.0752, -10031.1872)
  line L503 (-10069.6775, -10031.066) -> (-10067.9284, -10030.9775)
  ellipse E403 centre (-10072.8027, -10009.4797) end of major axis (-10072.6142, -10009.4561) minor radius 0.0959 (-10072.6139, -10009.4584) -> (-10072.81, -10009.384) ccw
  line L504 (-10072.6142, -10009.4561) -> (-10072.6108, -10009.4826)
  line L505 (-10072.5988, -10009.6576) -> (-10072.6139, -10009.4584)
  line L506 (-10070.181, -10009.3015) -> (-10070.1661, -10009.4975)
  line L507 (-10070.3476, -10009.6145) -> (-10071.2357, -10009.7146)
  line L508 (-10072.81, -10009.384) -> (-10074.2008, -10009.5408)
  line L509 (-10074.3823, -10009.6579) -> (-10074.3666, -10009.8642)
  line L510 (-10068.3379, -10010.0841) -> (-10068.4095, -10009.1432)
  line L511 (-10068.3261, -10010.1556) -> (-10068.3741, -10009.5246)
  ellipse E404 centre (-10074.1936, -10009.6366) end of major axis (-10074.3821, -10009.6602) minor radius 0.0959 (-10074.2008, -10009.5408) -> (-10074.3823, -10009.6579) ccw
  ellipse E405 centre (-10070.3549, -10009.5187) end of major axis (-10070.1663, -10009.4951) minor radius 0.0959 (-10070.3476, -10009.6145) -> (-10070.1661, -10009.4975) ccw
  ellipse E406 centre (-10068.295, -10010.4267) end of major axis (-10068.2501, -10010.8242) minor radius 0.0085 (-10068.3379, -10010.0841) -> (-10068.3319, -10010.1547) ccw
  line L512 (-10074.363, -10028.3302) -> (-10074.3697, -10028.4328)
  line L513 (-10068.3992, -10028.957) -> (-10068.3499, -10028.2048)
  line L514 (-10068.5335, -10028.105) -> (-10068.6667, -10028.09)
  line L515 (-10068.3708, -10028.6417) -> (-10068.3333, -10028.0692)
  line L516 (-10072.6014, -10028.6322) -> (-10072.5951, -10028.5368)
  line L517 (-10071.1849, -10028.4716) -> (-10070.3452, -10028.5664)
  line L518 (-10070.1616, -10028.6661) -> (-10070.1773, -10028.9056)
  ellipse E407 centre (-10072.557, -10028.2707) end of major axis (-10072.6019, -10028.6682) minor radius 0.0085 (-10072.6014, -10028.6322) -> (-10072.6026, -10028.6593) ccw
  ellipse E408 centre (-10070.133, -10028.5441) end of major axis (-10070.1778, -10028.9416) minor radius 0.0085 (-10070.1773, -10028.9056) -> (-10070.1778, -10028.9416) ccw
  ellipse E409 centre (-10070.3503, -10028.6448) end of major axis (-10070.1618, -10028.6679) minor radius 0.0785 (-10070.1616, -10028.6661) -> (-10070.3452, -10028.5664) ccw
  ellipse E410 centre (-10068.5387, -10028.1835) end of major axis (-10068.3501, -10028.2066) minor radius 0.0785 (-10068.3499, -10028.2048) -> (-10068.5335, -10028.105) ccw
  ellipse E411 centre (-10068.522, -10028.0479) end of major axis (-10068.3335, -10028.071) minor radius 0.0785 (-10068.3333, -10028.0692) -> (-10068.343, -10028.041) ccw
  ellipse E412 centre (-10074.3254, -10028.0713) end of major axis (-10074.3702, -10028.4688) minor radius 0.0085 (-10074.3697, -10028.4328) -> (-10074.3702, -10028.4688) ccw
  line L519 (-10074.3702, -10028.4688) -> (-10074.3427, -10028.4719)
  line L520 (-10070.1778, -10028.9416) -> (-10070.1673, -10028.9428)
  ellipse E413 centre (-10072.2464, -10007.1264) end of major axis (-10072.0671, -10007.1893) minor radius 0.1599 (-10072.0597, -10007.1359) -> (-10072.1007, -10007.0384) ccw
  ellipse E414 centre (-10072.2732, -10007.2029) end of major axis (-10072.0939, -10007.2658) minor radius 0.1599 (-10072.0865, -10007.2124) -> (-10072.1217, -10007.122) ccw
  ellipse E415 centre (-10072.2898, -10007.0593) end of major axis (-10072.1001, -10007.0484) minor radius 0.0969 (-10072.1031, -10007.0687) -> (-10072.1001, -10007.0484) ccw
  ellipse E416 centre (-10072.2972, -10006.9305) end of major axis (-10072.1075, -10006.9196) minor radius 0.0969 (-10072.1105, -10006.9399) -> (-10072.2632, -10006.8336) ccw
  ellipse E417 centre (-10069.5261, -10007.0706) end of major axis (-10069.7158, -10007.0815) minor radius 0.0969 (-10069.4922, -10006.9737) -> (-10069.7128, -10007.0612) ccw
  line L521 (-10072.1075, -10006.9196) -> (-10072.1001, -10007.0484)
  line L522 (-10072.0812, -10007.3046) -> (-10072.0865, -10007.2124)
  line L523 (-10072.0597, -10007.1359) -> (-10072.0473, -10007.3515)
  line L524 (-10072.2214, -10007.2562) -> (-10072.1105, -10006.9399)
  line L525 (-10072.1031, -10007.0687) -> (-10072.1932, -10007.3257)
  line L526 (-10072.5003, -10008.0519) -> (-10072.3966, -10007.756)
  line L527 (-10072.1759, -10007.6686) -> (-10070.1517, -10007.7709)
  line L528 (-10069.9989, -10007.8772) -> (-10070.1027, -10008.1731)
  line L529 (-10069.7128, -10007.0612) -> (-10069.8237, -10007.3774)
  line L530 (-10070.0444, -10007.4649) -> (-10072.0686, -10007.3625)
  ellipse E418 centre (-10072.4806, -10008.3953) end of major axis (-10072.4604, -10007.9959) minor radius 0.0715 (-10072.5003, -10008.0519) -> (-10072.5547, -10008.4848) ccw
  ellipse E419 centre (-10072.4806, -10008.3953) end of major axis (-10072.4932, -10008.645) minor radius 0.0447 (-10072.4929, -10008.1807) -> (-10072.5253, -10008.3944) ccw
  line L531 (-10072.3892, -10007.8848) -> (-10072.4929, -10008.1807)
  ellipse E420 centre (-10070.0829, -10008.5166) end of major axis (-10070.1031, -10008.9161) minor radius 0.0715 (-10070.1027, -10008.1731) -> (-10070.1571, -10008.6084) ccw
  line L532 (-10070.1443, -10007.8997) -> (-10072.1685, -10007.7974)
  line L533 (-10070.3582, -10009.3011) -> (-10070.6637, -10009.2856)
  line L534 (-10071.8828, -10009.224) -> (-10072.313, -10009.2022)
  line L535 (-10067.9398, -10007.422) -> (-10067.8805, -10008.4527)
  line L536 (-10067.8492, -10008.4543) -> (-10067.9129, -10007.3455)
  ellipse E421 centre (-10068.1265, -10007.4126) end of major axis (-10067.9472, -10007.4754) minor radius 0.1599 (-10067.9398, -10007.422) -> (-10067.975, -10007.3316) ccw
  ellipse E422 centre (-10068.0996, -10007.3361) end of major axis (-10067.9203, -10007.3989) minor radius 0.1599 (-10067.9129, -10007.3455) -> (-10067.9539, -10007.248) ccw
  line L537 (-10072.2632, -10006.8336) -> (-10073.6389, -10006.764)
  line L538 (-10073.8596, -10006.8515) -> (-10074.2494, -10007.9634)
  line L539 (-10068.3536, -10008.2615) -> (-10067.9637, -10007.1496)
  line L540 (-10068.1165, -10007.0432) -> (-10069.4922, -10006.9737)
  line L541 (-10068.3462, -10008.3903) -> (-10067.9563, -10007.2784)
  ellipse E423 centre (-10073.6729, -10006.861) end of major axis (-10073.8626, -10006.8719) minor radius 0.0969 (-10073.6389, -10006.764) -> (-10073.8596, -10006.8515) ccw
  ellipse E424 centre (-10068.1504, -10007.1402) end of major axis (-10067.9608, -10007.1292) minor radius 0.0969 (-10067.9637, -10007.1496) -> (-10068.1165, -10007.0432) ccw
  ellipse E425 centre (-10068.143, -10007.269) end of major axis (-10067.9533, -10007.2581) minor radius 0.0969 (-10067.9563, -10007.2784) -> (-10067.9533, -10007.2581) ccw
  line L542 (-10067.9608, -10007.1292) -> (-10067.9533, -10007.2581)
  ellipse E426 centre (-10072.2099, -10007.7655) end of major axis (-10072.3996, -10007.7764) minor radius 0.0969 (-10072.1759, -10007.6686) -> (-10072.3966, -10007.756) ccw
  ellipse E427 centre (-10070.1856, -10007.8678) end of major axis (-10069.996, -10007.8569) minor radius 0.0969 (-10069.9989, -10007.8772) -> (-10070.1517, -10007.7709) ccw
  ellipse E428 centre (-10070.0104, -10007.368) end of major axis (-10069.8207, -10007.3571) minor radius 0.0969 (-10070.0444, -10007.4649) -> (-10069.8237, -10007.3774) ccw
  ellipse E429 centre (-10072.0347, -10007.2656) end of major axis (-10072.2243, -10007.2765) minor radius 0.0969 (-10072.2214, -10007.2562) -> (-10072.0686, -10007.3625) ccw
  ellipse E430 centre (-10072.2025, -10007.8943) end of major axis (-10072.3922, -10007.9052) minor radius 0.0969 (-10072.1685, -10007.7974) -> (-10072.3892, -10007.8848) ccw
  ellipse E431 centre (-10072.3139, -10008.9616) end of major axis (-10072.4932, -10008.8988) minor radius 0.1599 (-10072.3353, -10009.121) -> (-10072.3248, -10009.1228) ccw
  ellipse E432 centre (-10072.3407, -10009.0382) end of major axis (-10072.1614, -10009.101) minor radius 0.1599 (-10072.3635, -10009.1973) -> (-10072.3483, -10009.1998) ccw
  ellipse E433 centre (-10070.3165, -10009.1405) end of major axis (-10070.1372, -10009.2034) minor radius 0.1599 (-10070.2512, -10009.2989) -> (-10070.1854, -10009.2687) ccw
  ellipse E434 centre (-10070.2896, -10009.064) end of major axis (-10070.4689, -10009.0011) minor radius 0.1599 (-10070.2361, -10009.2247) -> (-10070.1897, -10009.2107) ccw
  ellipse E435 centre (-10070.1782, -10007.9966) end of major axis (-10069.9886, -10007.9857) minor radius 0.0969 (-10070.0197, -10007.9365) -> (-10070.1443, -10007.8997) ccw
  line L543 (-10068.3388, -10009.424) -> (-10068.3749, -10008.7949)
  line L544 (-10068.4003, -10008.897) -> (-10068.3887, -10009.0976)
  line L545 (-10068.3686, -10009.4481) -> (-10068.3653, -10009.5052)
  ellipse E436 centre (-10068.3338, -10008.605) end of major axis (-10068.3212, -10008.3553) minor radius 0.0447 (-10068.3462, -10008.3903) -> (-10068.3719, -10008.5218) ccw
  ellipse E437 centre (-10074.2297, -10008.3069) end of major axis (-10074.2499, -10008.7064) minor radius 0.0715 (-10074.2494, -10007.9634) -> (-10074.3035, -10008.4503) ccw
  ellipse E438 centre (-10068.3338, -10008.605) end of major axis (-10068.354, -10009.0045) minor radius 0.0715 (-10068.3536, -10008.2615) -> (-10068.4065, -10008.6307) ccw
  ellipse E439 centre (-10072.7769, -10029.133) end of major axis (-10072.5961, -10029.0746) minor radius 0.168 (-10072.7891, -10029.3032) -> (-10072.5893, -10029.1318) ccw
  ellipse E440 centre (-10072.7554, -10029.1997) end of major axis (-10072.5746, -10029.1413) minor radius 0.168 (-10072.6445, -10029.3296) -> (-10072.5677, -10029.1985) ccw
  ellipse E441 centre (-10069.9705, -10029.1814) end of major axis (-10070.1513, -10029.2398) minor radius 0.168 (-10070.1513, -10029.2398) -> (-10070.1111, -10029.3032) ccw
  ellipse E442 centre (-10072.7619, -10029.3886) end of major axis (-10072.5724, -10029.4022) minor radius 0.0836 (-10072.5742, -10029.3874) -> (-10072.7892, -10029.3041) ccw
  ellipse E443 centre (-10072.7715, -10029.5229) end of major axis (-10072.582, -10029.5365) minor radius 0.0836 (-10072.5839, -10029.5217) -> (-10072.7988, -10029.4384) ccw
  ellipse E444 centre (-10069.9866, -10029.5046) end of major axis (-10070.1762, -10029.491) minor radius 0.0836 (-10070.0139, -10029.4201) -> (-10070.1743, -10029.5058) ccw
  ellipse E445 centre (-10069.9921, -10029.1147) end of major axis (-10070.1729, -10029.1731) minor radius 0.168 (-10070.1797, -10029.1159) -> (-10070.0043, -10029.2848) ccw
  ellipse E446 centre (-10069.977, -10029.3702) end of major axis (-10070.1665, -10029.3567) minor radius 0.0836 (-10070.0043, -10029.2857) -> (-10070.1665, -10029.3567) ccw
  line L546 (-10070.1729, -10029.1731) -> (-10070.1513, -10029.2398)
  line L547 (-10070.1665, -10029.3567) -> (-10070.1762, -10029.491)
  line L548 (-10072.5318, -10028.6979) -> (-10072.5677, -10029.1985)
  line L549 (-10072.5893, -10029.1318) -> (-10072.5534, -10028.6311)
  line L550 (-10072.4948, -10029.7975) -> (-10072.499, -10029.7843)
  line L551 (-10072.4995, -10029.783) -> (-10072.5839, -10029.5217)
  line L552 (-10072.5742, -10029.3874) -> (-10072.5193, -10029.5576)
  line L553 (-10070.1743, -10029.5058) -> (-10070.1245, -10029.66)
  line L554 (-10070.2455, -10029.8674) -> (-10071.5141, -10029.8757)
  line L555 (-10071.9554, -10029.8786) -> (-10072.2798, -10029.8808)
  line L556 (-10070.1613, -10028.8588) -> (-10070.1797, -10029.1159)
  line L557 (-10072.2702, -10029.7464) -> (-10072.0138, -10029.7448)
  line L558 (-10070.5805, -10029.7353) -> (-10070.2359, -10029.733)
  ellipse E447 centre (-10074.1379, -10029.2089) end of major axis (-10074.3187, -10029.2673) minor radius 0.168 (-10074.3187, -10029.2673) -> (-10074.2785, -10029.3307) ccw
  ellipse E448 centre (-10068.5879, -10029.1723) end of major axis (-10068.4071, -10029.1139) minor radius 0.168 (-10068.477, -10029.3021) -> (-10068.4003, -10029.171) ccw
  ellipse E449 centre (-10068.6095, -10029.1056) end of major axis (-10068.4287, -10029.0472) minor radius 0.168 (-10068.6217, -10029.2757) -> (-10068.4219, -10029.1043) ccw
  ellipse E450 centre (-10074.1595, -10029.1421) end of major axis (-10074.3403, -10029.2005) minor radius 0.168 (-10074.3471, -10029.1434) -> (-10074.1717, -10029.3123) ccw
  line L559 (-10074.3187, -10029.2673) -> (-10074.3403, -10029.2005)
  line L560 (-10068.4003, -10029.171) -> (-10068.3869, -10028.9841)
  line L561 (-10068.3682, -10028.7233) -> (-10068.3415, -10028.3506)
  line L562 (-10068.6217, -10029.2757) -> (-10070.0043, -10029.2848)
  line L563 (-10068.4092, -10028.9276) -> (-10068.4219, -10029.1043)
  line L564 (-10074.3471, -10029.1434) -> (-10074.315, -10028.6954)
  line L565 (-10072.7891, -10029.3032) -> (-10074.1717, -10029.3123)
  ellipse E451 centre (-10072.3442, -10028.6966) end of major axis (-10072.525, -10028.755) minor radius 0.168 (-10072.4372, -10028.5552) -> (-10072.5318, -10028.6979) ccw
  ellipse E452 centre (-10070.2728, -10029.7829) end of major axis (-10070.0833, -10029.7964) minor radius 0.0836 (-10070.2455, -10029.8674) -> (-10070.1556, -10029.8555) ccw
  ellipse E453 centre (-10072.3071, -10029.7963) end of major axis (-10072.4967, -10029.7827) minor radius 0.0836 (-10072.4948, -10029.7975) -> (-10072.4873, -10029.812) ccw